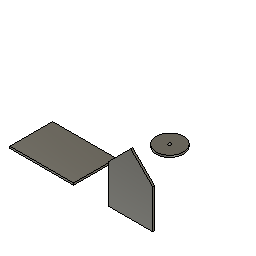
1stLesson(ExtrudeWheelRectangleBaseHole) v1 (Autodesk Fusion 360 design; units mm, degrees)
Autodesk Fusion 360 part; units mm, degrees
sketch "Sketch1" plane through (0, 0, 0) normal (0, 0, 1) x (1, 0, 0)
  line L0 (6.8128, 0.929) -> (88.8128, 0.929)
  line L1 (88.8128, 0.929) -> (88.8128, 55.929)
  line L2 (88.8128, 55.929) -> (6.8128, 55.929)
  line L3 (6.8128, 55.929) -> (6.8128, 0.929)
  dimension "d1" = 82
  dimension "d2" = 55
  constraint horizontal L0
  constraint vertical L1
  constraint horizontal L2
  constraint vertical L3
  measures "d1" distance of L0.start L0.end
  measures "d2" distance of L0.start L2.end
extrude "Extrude1" add sketch "Sketch1" along normal blind 2.5 makes body 1
sketch "Sketch2" plane through (0, 0, 2.5) normal (0, 0, 1) x (-1, 0, 0)
  line L0 (-6.8128, -55.929) -> (-6.8128, -0.929)
  line L1 (-6.8128, -0.929) -> (-88.8128, -0.929)
  line L2 (-88.8128, -0.929) -> (-88.8128, -55.929)
  line L3 (-88.8128, -55.929) -> (-6.8128, -55.929)
  circle A0 centre (-109.9836, -103.7173) radius 17.5
  dimension "d5" = 35
  measures "d5" diameter of A0
extrude "Extrude2" add sketch "Sketch2" along normal blind 2.5 separate body contours A0 makes body 2
sketch "Sketch3" plane through (0, 0, 5) normal (0, 0, 1) x (-1, 0, 0)
  circle A0 centre (-109.9836, -103.7173) radius 17.5
  circle A1 centre (-109.9836, -103.7173) radius 2
  dimension "d8" = 4
  constraint concentric A0 A1
  measures "d8" diameter of A1
extrude "Extrude3" cut sketch "Sketch3" against normal blind 19 contours A1 bodies 2
sketch "Sketch4" plane through (0, 0, 0) normal (0, 1, 0) x (1, 0, 0)
  line L0 (135, 0) -> (135, -50)
  line L1 (135, -50) -> (163.2843, -78.2843)
  line L2 (135, -50) -> (175, -50) construction
  line L3 (163.2843, -78.2843) -> (191.5685, -50)
  line L4 (163.2843, -78.2843) -> (203.2843, -78.2843) construction
  line L5 (191.5685, -50) -> (191.5685, 0)
  line L6 (191.5685, 0) -> (135, 0)
  dimension "d11" = 50
  dimension "d12" = 40
  dimension "d13" = 45
  dimension "d14" = 45
  dimension "d15" = 40
  dimension "d16" = 50
  constraint vertical L0
  constraint horizontal L2
  constraint horizontal L4
  constraint vertical L5
  measures "d11" distance of L0.start L0.end
  measures "d12" distance of L0.end L1.end
  measures "d13" angle of L1 L2
  measures "d14" angle of L3 L4
  measures "d15" distance of L1.end L3.end
  measures "d16" distance of L3.end L5.end
extrude "Extrude4" add sketch "Sketch4" along normal blind 2.5 separate body makes body 3
